Autodesk Fusion 360 part; units mm, degrees
(part 3 of 3)
  spline S32 degree 5 poles (-6.114, -23.4187) (-6.116, -23.4266) (-6.12, -23.4424) (-6.1254, -23.4662) (-6.1316, -23.4981) (-6.138, -23.5383) (-6.1434, -23.5788) (-6.1482, -23.6193) (-6.1527, -23.6599) (-6.157, -23.7006) (-6.1611, -23.7414) (-6.1648, -23.7822) (-6.1682, -23.8231) (-6.1711, -23.864) (-6.1735, -23.9051) (-6.1755, -23.9463) (-6.1771, -23.9875) (-6.1784, -24.0288) (-6.1795, -24.0701) (-6.1802, -24.1115) (-6.1807, -24.1529) (-6.181, -24.1944) (-6.1809, -24.2359) (-6.1806, -24.2775) (-6.18, -24.3191) (-6.1791, -24.3608) (-6.178, -24.4025) (-6.1765, -24.4442) (-6.1749, -24.486) (-6.173, -24.5279) (-6.1709, -24.5697) (-6.1685, -24.6116) (-6.1659, -24.6535) (-6.1631, -24.6955) (-6.16, -24.7375) (-6.1568, -24.7795) (-6.1532, -24.8215) (-6.1495, -24.8636) (-6.1456, -24.9057) (-6.1414, -24.9479) (-6.1371, -24.99) (-6.1325, -25.0322) (-6.1277, -25.0744) (-6.1227, -25.1166) (-6.1175, -25.1589) (-6.1121, -25.2012) (-6.1065, -25.2435) (-6.1007, -25.2858) (-6.0947, -25.3281) (-6.0886, -25.3705) (-6.0822, -25.4128) (-6.0756, -25.4552) (-6.0689, -25.4976) (-6.0619, -25.5401) (-6.0548, -25.5825) (-6.0475, -25.6249) (-6.04, -25.6674) (-6.0323, -25.7099) (-6.0244, -25.7524) (-6.0164, -25.7949) (-6.0081, -25.8374) (-5.9997, -25.88) (-5.9911, -25.9225) (-5.9824, -25.9651) (-5.9734, -26.0076) (-5.9643, -26.0502) (-5.9551, -26.0928) (-5.9456, -26.1354) (-5.936, -26.178) (-5.9262, -26.2206) (-5.9162, -26.2632) (-5.9081, -26.2973) (-5.9019, -26.3229) (-5.8978, -26.3399) (-5.8957, -26.3484) knots 0 0 0 0 0 0 0.01428571 0.02857143 0.04285714 0.05714286 0.07142857 0.08571429 0.1 0.11428571 0.12857143 0.14285714 0.15714286 0.17142857 0.18571429 0.2 0.21428571 0.22857143 0.24285714 0.25714286 0.27142857 0.28571429 0.3 0.31428571 0.32857143 0.34285714 0.35714286 0.37142857 0.38571429 0.4 0.41428571 0.42857143 0.44285714 0.45714286 0.47142857 0.48571429 0.5 0.51428571 0.52857143 0.54285714 0.55714286 0.57142857 0.58571429 0.6 0.61428571 0.62857143 0.64285714 0.65714286 0.67142857 0.68571429 0.7 0.71428571 0.72857143 0.74285714 0.75714286 0.77142857 0.78571429 0.8 0.81428571 0.82857143 0.84285714 0.85714286 0.87142857 0.88571429 0.9 0.91428571 0.92857143 0.94285714 0.95714286 0.97142857 0.98571429 1 1 1 1 1 1
  arc A66 (-5.8957, -26.3484) -> (-4.2178, -26.6685) centre (0, 0) ccw
  spline S33 degree 5 poles (-2.9364, -24.0249) (-2.9374, -24.033) (-2.9395, -24.0491) (-2.9433, -24.0732) (-2.9493, -24.1052) (-2.9581, -24.1449) (-2.9679, -24.1845) (-2.9784, -24.224) (-2.9891, -24.2634) (-3.0001, -24.3028) (-3.0114, -24.3422) (-3.0229, -24.3815) (-3.0348, -24.4208) (-3.0472, -24.46) (-3.0601, -24.499) (-3.0734, -24.538) (-3.087, -24.577) (-3.101, -24.6158) (-3.1153, -24.6546) (-3.1298, -24.6934) (-3.1446, -24.7321) (-3.1596, -24.7708) (-3.1749, -24.8094) (-3.1905, -24.8479) (-3.2064, -24.8864) (-3.2226, -24.9248) (-3.239, -24.9631) (-3.2557, -25.0014) (-3.2726, -25.0397) (-3.2898, -25.0779) (-3.3072, -25.116) (-3.3248, -25.1541) (-3.3426, -25.1921) (-3.3607, -25.2301) (-3.379, -25.268) (-3.3975, -25.3058) (-3.4163, -25.3436) (-3.4352, -25.3814) (-3.4544, -25.4191) (-3.4738, -25.4567) (-3.4934, -25.4943) (-3.5131, -25.5319) (-3.5331, -25.5694) (-3.5533, -25.6068) (-3.5737, -25.6442) (-3.5943, -25.6815) (-3.615, -25.7187) (-3.636, -25.7559) (-3.6571, -25.7931) (-3.6785, -25.8302) (-3.7, -25.8673) (-3.7217, -25.9043) (-3.7436, -25.9412) (-3.7657, -25.9781) (-3.7879, -26.0149) (-3.8104, -26.0517) (-3.833, -26.0884) (-3.8558, -26.1251) (-3.8787, -26.1617) (-3.9019, -26.1983) (-3.9252, -26.2348) (-3.9486, -26.2712) (-3.9723, -26.3076) (-3.9961, -26.344) (-4.0201, -26.3802) (-4.0442, -26.4165) (-4.0685, -26.4527) (-4.093, -26.4888) (-4.1176, -26.5248) (-4.1424, -26.5608) (-4.1674, -26.5968) (-4.1875, -26.6255) (-4.2026, -26.647) (-4.2127, -26.6614) (-4.2178, -26.6685) knots 0 0 0 0 0 0 0.01428571 0.02857143 0.04285714 0.05714286 0.07142857 0.08571429 0.1 0.11428571 0.12857143 0.14285714 0.15714286 0.17142857 0.18571429 0.2 0.21428571 0.22857143 0.24285714 0.25714286 0.27142857 0.28571429 0.3 0.31428571 0.32857143 0.34285714 0.35714286 0.37142857 0.38571429 0.4 0.41428571 0.42857143 0.44285714 0.45714286 0.47142857 0.48571429 0.5 0.51428571 0.52857143 0.54285714 0.55714286 0.57142857 0.58571429 0.6 0.61428571 0.62857143 0.64285714 0.65714286 0.67142857 0.68571429 0.7 0.71428571 0.72857143 0.74285714 0.75714286 0.77142857 0.78571429 0.8 0.81428571 0.82857143 0.84285714 0.85714286 0.87142857 0.88571429 0.9 0.91428571 0.92857143 0.94285714 0.95714286 0.97142857 0.98571429 1 1 1 1 1 1
  line L33 (-2.9364, -24.0249) -> (-2.8541, -23.3538)
  arc A67 (-1.7825, -22.4786) -> (-2.8541, -23.3538) centre (-1.8615, -23.4755) ccw
  arc A68 (-1.7825, -22.4786) -> (-1.0489, -22.5248) centre (0, 0) ccw
  arc A69 (-0.0954, -23.5274) -> (-1.0489, -22.5248) centre (-1.0954, -23.5237) ccw
  line L34 (-0.0954, -23.5274) -> (-0.0979, -24.2035)
  spline S34 degree 5 poles (-0.0979, -24.2035) (-0.0979, -24.2116) (-0.0978, -24.2279) (-0.0971, -24.2523) (-0.0952, -24.2848) (-0.0914, -24.3253) (-0.0866, -24.3658) (-0.0812, -24.4063) (-0.0755, -24.4467) (-0.0695, -24.4872) (-0.0633, -24.5277) (-0.0568, -24.5682) (-0.0498, -24.6086) (-0.0425, -24.649) (-0.0346, -24.6894) (-0.0263, -24.7297) (-0.0176, -24.7701) (-0.0086, -24.8104) (0.0007, -24.8507) (0.0102, -24.891) (0.02, -24.9312) (0.0301, -24.9714) (0.0405, -25.0117) (0.0511, -25.0518) (0.0621, -25.092) (0.0733, -25.1321) (0.0848, -25.1722) (0.0965, -25.2123) (0.1085, -25.2524) (0.1208, -25.2924) (0.1332, -25.3324) (0.1459, -25.3724) (0.1589, -25.4124) (0.172, -25.4523) (0.1855, -25.4922) (0.1991, -25.5321) (0.2129, -25.572) (0.227, -25.6118) (0.2413, -25.6516) (0.2558, -25.6914) (0.2705, -25.7311) (0.2854, -25.7709) (0.3006, -25.8105) (0.3159, -25.8502) (0.3314, -25.8898) (0.3472, -25.9294) (0.3631, -25.969) (0.3792, -26.0086) (0.3956, -26.0481) (0.4121, -26.0876) (0.4288, -26.127) (0.4457, -26.1664) (0.4628, -26.2058) (0.4801, -26.2452) (0.4975, -26.2845) (0.5152, -26.3238) (0.533, -26.3631) (0.551, -26.4023) (0.5692, -26.4415) (0.5876, -26.4807) (0.6061, -26.5199) (0.6248, -26.559) (0.6437, -26.598) (0.6628, -26.6371) (0.6821, -26.6761) (0.7015, -26.715) (0.721, -26.754) (0.7408, -26.7929) (0.7607, -26.8318) (0.7808, -26.8706) (0.8011, -26.9094) (0.8174, -26.9404) (0.8297, -26.9636) (0.838, -26.9791) (0.8421, -26.9869) knots 0 0 0 0 0 0 0.01428571 0.02857143 0.04285714 0.05714286 0.07142857 0.08571429 0.1 0.11428571 0.12857143 0.14285714 0.15714286 0.17142857 0.18571429 0.2 0.21428571 0.22857143 0.24285714 0.25714286 0.27142857 0.28571429 0.3 0.31428571 0.32857143 0.34285714 0.35714286 0.37142857 0.38571429 0.4 0.41428571 0.42857143 0.44285714 0.45714286 0.47142857 0.48571429 0.5 0.51428571 0.52857143 0.54285714 0.55714286 0.57142857 0.58571429 0.6 0.61428571 0.62857143 0.64285714 0.65714286 0.67142857 0.68571429 0.7 0.71428571 0.72857143 0.74285714 0.75714286 0.77142857 0.78571429 0.8 0.81428571 0.82857143 0.84285714 0.85714286 0.87142857 0.88571429 0.9 0.91428571 0.92857143 0.94285714 0.95714286 0.97142857 0.98571429 1 1 1 1 1 1
  arc A70 (0.8421, -26.9869) -> (2.5469, -26.8796) centre (0, 0) ccw
  spline S35 degree 5 poles (3.1306, -24.0004) (3.1317, -24.0084) (3.1336, -24.0246) (3.136, -24.0489) (3.1381, -24.0813) (3.1394, -24.122) (3.1398, -24.1628) (3.1395, -24.2036) (3.1388, -24.2445) (3.138, -24.2854) (3.1369, -24.3264) (3.1355, -24.3673) (3.1337, -24.4083) (3.1315, -24.4493) (3.1287, -24.4904) (3.1256, -24.5314) (3.122, -24.5725) (3.1181, -24.6137) (3.1139, -24.6548) (3.1095, -24.696) (3.1048, -24.7371) (3.0999, -24.7783) (3.0946, -24.8195) (3.0891, -24.8607) (3.0833, -24.9019) (3.0772, -24.9431) (3.0708, -24.9844) (3.0642, -25.0256) (3.0573, -25.0669) (3.0502, -25.1081) (3.0428, -25.1494) (3.0352, -25.1907) (3.0274, -25.2319) (3.0193, -25.2732) (3.011, -25.3145) (3.0025, -25.3557) (2.9938, -25.397) (2.9848, -25.4383) (2.9756, -25.4796) (2.9662, -25.5209) (2.9566, -25.5621) (2.9468, -25.6034) (2.9367, -25.6447) (2.9265, -25.686) (2.916, -25.7272) (2.9054, -25.7685) (2.8945, -25.8098) (2.8835, -25.851) (2.8722, -25.8923) (2.8608, -25.9335) (2.8492, -25.9747) (2.8373, -26.016) (2.8253, -26.0572) (2.8131, -26.0984) (2.8007, -26.1396) (2.7881, -26.1808) (2.7754, -26.222) (2.7624, -26.2632) (2.7493, -26.3044) (2.736, -26.3456) (2.7225, -26.3867) (2.7088, -26.4279) (2.695, -26.469) (2.6809, -26.5101) (2.6667, -26.5512) (2.6523, -26.5923) (2.6378, -26.6334) (2.6231, -26.6745) (2.6082, -26.7155) (2.5931, -26.7566) (2.5779, -26.7976) (2.5656, -26.8304) (2.5563, -26.855) (2.55, -26.8714) (2.5469, -26.8796) knots 0 0 0 0 0 0 0.01428571 0.02857143 0.04285714 0.05714286 0.07142857 0.08571429 0.1 0.11428571 0.12857143 0.14285714 0.15714286 0.17142857 0.18571429 0.2 0.21428571 0.22857143 0.24285714 0.25714286 0.27142857 0.28571429 0.3 0.31428571 0.32857143 0.34285714 0.35714286 0.37142857 0.38571429 0.4 0.41428571 0.42857143 0.44285714 0.45714286 0.47142857 0.48571429 0.5 0.51428571 0.52857143 0.54285714 0.55714286 0.57142857 0.58571429 0.6 0.61428571 0.62857143 0.64285714 0.65714286 0.67142857 0.68571429 0.7 0.71428571 0.72857143 0.74285714 0.75714286 0.77142857 0.78571429 0.8 0.81428571 0.82857143 0.84285714 0.85714286 0.87142857 0.88571429 0.9 0.91428571 0.92857143 0.94285714 0.95714286 0.97142857 0.98571429 1 1 1 1 1 1
  line L35 (3.1306, -24.0004) -> (3.0434, -23.3299)
  arc A71 (3.8637, -22.2157) -> (3.0434, -23.3299) centre (4.0351, -23.2009) ccw
  arc A72 (3.8637, -22.2157) -> (4.5857, -22.078) centre (0, 0) ccw
  arc A73 (5.7586, -22.8119) -> (4.5857, -22.078) centre (4.7891, -23.0571) ccw
  line L36 (5.7586, -22.8119) -> (5.9243, -23.4674)
  spline S36 degree 5 poles (5.9243, -23.4674) (5.9263, -23.4753) (5.9305, -23.4911) (5.9372, -23.5145) (5.9472, -23.5455) (5.9609, -23.5838) (5.9756, -23.6218) (5.9909, -23.6597) (6.0066, -23.6975) (6.0224, -23.7352) (6.0385, -23.7728) (6.0549, -23.8104) (6.0716, -23.8479) (6.0888, -23.8852) (6.1065, -23.9223) (6.1246, -23.9594) (6.143, -23.9963) (6.1618, -24.0331) (6.1808, -24.0698) (6.2, -24.1064) (6.2195, -24.143) (6.2393, -24.1794) (6.2593, -24.2158) (6.2797, -24.2521) (6.3002, -24.2882) (6.3211, -24.3243) (6.3422, -24.3603) (6.3636, -24.3962) (6.3851, -24.432) (6.4069, -24.4678) (6.429, -24.5034) (6.4512, -24.539) (6.4737, -24.5745) (6.4964, -24.6099) (6.5193, -24.6452) (6.5424, -24.6805) (6.5657, -24.7156) (6.5893, -24.7507) (6.613, -24.7857) (6.637, -24.8206) (6.6611, -24.8555) (6.6854, -24.8902) (6.7099, -24.9249) (6.7347, -24.9595) (6.7596, -24.994) (6.7847, -25.0285) (6.8099, -25.0629) (6.8354, -25.0971) (6.861, -25.1314) (6.8869, -25.1655) (6.9129, -25.1996) (6.939, -25.2335) (6.9654, -25.2674) (6.9919, -25.3013) (7.0186, -25.335) (7.0455, -25.3687) (7.0725, -25.4023) (7.0997, -25.4358) (7.1271, -25.4693) (7.1546, -25.5027) (7.1823, -25.5359) (7.2102, -25.5692) (7.2382, -25.6023) (7.2664, -25.6354) (7.2947, -25.6684) (7.3232, -25.7013) (7.3518, -25.7341) (7.3806, -25.7669) (7.4096, -25.7996) (7.4387, -25.8322) (7.468, -25.8648) (7.4915, -25.8907) (7.5092, -25.9102) (7.5211, -25.9231) (7.527, -25.9296) knots 0 0 0 0 0 0 0.01428571 0.02857143 0.04285714 0.05714286 0.07142857 0.08571429 0.1 0.11428571 0.12857143 0.14285714 0.15714286 0.17142857 0.18571429 0.2 0.21428571 0.22857143 0.24285714 0.25714286 0.27142857 0.28571429 0.3 0.31428571 0.32857143 0.34285714 0.35714286 0.37142857 0.38571429 0.4 0.41428571 0.42857143 0.44285714 0.45714286 0.47142857 0.48571429 0.5 0.51428571 0.52857143 0.54285714 0.55714286 0.57142857 0.58571429 0.6 0.61428571 0.62857143 0.64285714 0.65714286 0.67142857 0.68571429 0.7 0.71428571 0.72857143 0.74285714 0.75714286 0.77142857 0.78571429 0.8 0.81428571 0.82857143 0.84285714 0.85714286 0.87142857 0.88571429 0.9 0.91428571 0.92857143 0.94285714 0.95714286 0.97142857 0.98571429 1 1 1 1 1 1
  arc A74 (7.527, -25.9296) -> (9.1516, -25.4017) centre (0, 0) ccw
  spline S37 degree 5 poles (9.0009, -22.4678) (9.0039, -22.4754) (9.0098, -22.4905) (9.0182, -22.5135) (9.0283, -22.5444) (9.0397, -22.5834) (9.0502, -22.6229) (9.06, -22.6625) (9.0696, -22.7022) (9.0789, -22.7421) (9.0881, -22.782) (9.0969, -22.822) (9.1054, -22.8621) (9.1134, -22.9024) (9.1209, -22.9429) (9.1281, -22.9834) (9.1349, -23.0241) (9.1413, -23.0649) (9.1475, -23.1058) (9.1535, -23.1468) (9.1592, -23.1878) (9.1646, -23.2289) (9.1698, -23.2701) (9.1747, -23.3114) (9.1793, -23.3528) (9.1836, -23.3942) (9.1877, -23.4358) (9.1915, -23.4774) (9.1951, -23.519) (9.1985, -23.5608) (9.2016, -23.6026) (9.2045, -23.6444) (9.2072, -23.6863) (9.2097, -23.7283) (9.2119, -23.7704) (9.2139, -23.8125) (9.2157, -23.8546) (9.2173, -23.8968) (9.2186, -23.9391) (9.2198, -23.9814) (9.2207, -24.0238) (9.2215, -24.0662) (9.222, -24.1087) (9.2224, -24.1512) (9.2225, -24.1938) (9.2225, -24.2364) (9.2222, -24.2791) (9.2218, -24.3218) (9.2211, -24.3645) (9.2203, -24.4073) (9.2193, -24.4501) (9.2181, -24.493) (9.2167, -24.5359) (9.2151, -24.5789) (9.2134, -24.6219) (9.2114, -24.6649) (9.2093, -24.708) (9.207, -24.7511) (9.2045, -24.7943) (9.2019, -24.8375) (9.199, -24.8807) (9.196, -24.9239) (9.1929, -24.9672) (9.1895, -25.0105) (9.186, -25.0539) (9.1823, -25.0973) (9.1784, -25.1407) (9.1743, -25.1841) (9.1701, -25.2276) (9.1658, -25.2711) (9.1612, -25.3146) (9.1574, -25.3494) (9.1545, -25.3756) (9.1526, -25.393) (9.1516, -25.4017) knots 0 0 0 0 0 0 0.01428571 0.02857143 0.04285714 0.05714286 0.07142857 0.08571429 0.1 0.11428571 0.12857143 0.14285714 0.15714286 0.17142857 0.18571429 0.2 0.21428571 0.22857143 0.24285714 0.25714286 0.27142857 0.28571429 0.3 0.31428571 0.32857143 0.34285714 0.35714286 0.37142857 0.38571429 0.4 0.41428571 0.42857143 0.44285714 0.45714286 0.47142857 0.48571429 0.5 0.51428571 0.52857143 0.54285714 0.55714286 0.57142857 0.58571429 0.6 0.61428571 0.62857143 0.64285714 0.65714286 0.67142857 0.68571429 0.7 0.71428571 0.72857143 0.74285714 0.75714286 0.77142857 0.78571429 0.8 0.81428571 0.82857143 0.84285714 0.85714286 0.87142857 0.88571429 0.9 0.91428571 0.92857143 0.94285714 0.95714286 0.97142857 0.98571429 1 1 1 1 1 1
  line L37 (9.0009, -22.4678) -> (8.7497, -21.84)
  arc A75 (9.2672, -20.5569) -> (8.7497, -21.84) centre (9.6782, -21.4685) ccw
  arc A76 (9.2672, -20.5569) -> (9.9322, -20.2439) centre (0, 0) ccw
  arc A77 (11.2508, -20.6632) -> (9.9322, -20.2439) centre (10.3727, -21.1417) ccw
  line L38 (11.2508, -20.6632) -> (11.5743, -21.2568)
  spline S38 degree 5 poles (11.5743, -21.2568) (11.5782, -21.264) (11.5862, -21.2782) (11.5985, -21.2992) (11.6159, -21.3267) (11.6387, -21.3604) (11.6624, -21.3936) (11.6867, -21.4265) (11.7112, -21.4592) (11.7359, -21.4918) (11.7609, -21.5243) (11.7861, -21.5566) (11.8116, -21.5887) (11.8375, -21.6205) (11.8639, -21.6521) (11.8906, -21.6835) (11.9176, -21.7147) (11.945, -21.7457) (11.9725, -21.7765) (12.0003, -21.8072) (12.0283, -21.8377) (12.0565, -21.8681) (12.0849, -21.8984) (12.1136, -21.9285) (12.1426, -21.9584) (12.1717, -21.9881) (12.2011, -22.0178) (12.2307, -22.0472) (12.2605, -22.0766) (12.2906, -22.1057) (12.3208, -22.1348) (12.3512, -22.1637) (12.3817, -22.1925) (12.4125, -22.2212) (12.4435, -22.2497) (12.4747, -22.2781) (12.506, -22.3063) (12.5375, -22.3344) (12.5692, -22.3624) (12.6011, -22.3903) (12.6331, -22.418) (12.6653, -22.4457) (12.6977, -22.4732) (12.7303, -22.5005) (12.763, -22.5278) (12.7958, -22.5549) (12.8289, -22.5819) (12.8621, -22.6088) (12.8954, -22.6355) (12.9289, -22.6622) (12.9626, -22.6887) (12.9964, -22.7151) (13.0303, -22.7414) (13.0644, -22.7676) (13.0987, -22.7936) (13.1331, -22.8196) (13.1676, -22.8454) (13.2023, -22.8711) (13.2371, -22.8967) (13.2721, -22.9222) (13.3072, -22.9475) (13.3424, -22.9728) (13.3778, -22.9979) (13.4133, -23.0229) (13.449, -23.0478) (13.4848, -23.0726) (13.5207, -23.0973) (13.5567, -23.1219) (13.5929, -23.1464) (13.6292, -23.1707) (13.6657, -23.195) (13.6949, -23.2143) (13.7169, -23.2287) (13.7316, -23.2383) (13.739, -23.2431) knots 0 0 0 0 0 0 0.01428571 0.02857143 0.04285714 0.05714286 0.07142857 0.08571429 0.1 0.11428571 0.12857143 0.14285714 0.15714286 0.17142857 0.18571429 0.2 0.21428571 0.22857143 0.24285714 0.25714286 0.27142857 0.28571429 0.3 0.31428571 0.32857143 0.34285714 0.35714286 0.37142857 0.38571429 0.4 0.41428571 0.42857143 0.44285714 0.45714286 0.47142857 0.48571429 0.5 0.51428571 0.52857143 0.54285714 0.55714286 0.57142857 0.58571429 0.6 0.61428571 0.62857143 0.64285714 0.65714286 0.67142857 0.68571429 0.7 0.71428571 0.72857143 0.74285714 0.75714286 0.77142857 0.78571429 0.8 0.81428571 0.82857143 0.84285714 0.85714286 0.87142857 0.88571429 0.9 0.91428571 0.92857143 0.94285714 0.95714286 0.97142857 0.98571429 1 1 1 1 1 1
  arc A78 (13.739, -23.2431) -> (15.1812, -22.3278) centre (0, 0) ccw
  spline S39 degree 5 poles (14.3057, -19.5235) (14.3105, -19.5301) (14.3199, -19.5433) (14.3337, -19.5634) (14.3512, -19.5908) (14.372, -19.6259) (14.3919, -19.6614) (14.4113, -19.6974) (14.4305, -19.7335) (14.4494, -19.7697) (14.4682, -19.8061) (14.4867, -19.8427) (14.5049, -19.8795) (14.5227, -19.9165) (14.5401, -19.9538) (14.5571, -19.9913) (14.5737, -20.0291) (14.5901, -20.067) (14.6063, -20.105) (14.6223, -20.1432) (14.638, -20.1815) (14.6535, -20.22) (14.6687, -20.2586) (14.6837, -20.2974) (14.6985, -20.3363) (14.713, -20.3754) (14.7273, -20.4146) (14.7413, -20.454) (14.7552, -20.4934) (14.7688, -20.533) (14.7822, -20.5727) (14.7955, -20.6125) (14.8085, -20.6524) (14.8213, -20.6925) (14.8339, -20.7327) (14.8463, -20.7729) (14.8586, -20.8133) (14.8706, -20.8538) (14.8824, -20.8944) (14.8941, -20.9351) (14.9055, -20.9759) (14.9168, -21.0168) (14.9279, -21.0578) (14.9388, -21.0989) (14.9495, -21.1401) (14.9601, -21.1814) (14.9704, -21.2228) (14.9806, -21.2643) (14.9907, -21.3059) (15.0005, -21.3475) (15.0102, -21.3893) (15.0197, -21.4311) (15.029, -21.473) (15.0382, -21.515) (15.0471, -21.5571) (15.056, -21.5993) (15.0646, -21.6415) (15.0731, -21.6838) (15.0814, -21.7262) (15.0896, -21.7687) (15.0976, -21.8113) (15.1055, -21.8539) (15.1131, -21.8966) (15.1207, -21.9394) (15.128, -21.9823) (15.1352, -22.0252) (15.1423, -22.0683) (15.1491, -22.1113) (15.1559, -22.1545) (15.1625, -22.1977) (15.1689, -22.241) (15.1739, -22.2757) (15.1776, -22.3017) (15.18, -22.3191) (15.1812, -22.3278) knots 0 0 0 0 0 0 0.01428571 0.02857143 0.04285714 0.05714286 0.07142857 0.08571429 0.1 0.11428571 0.12857143 0.14285714 0.15714286 0.17142857 0.18571429 0.2 0.21428571 0.22857143 0.24285714 0.25714286 0.27142857 0.28571429 0.3 0.31428571 0.32857143 0.34285714 0.35714286 0.37142857 0.38571429 0.4 0.41428571 0.42857143 0.44285714 0.45714286 0.47142857 0.48571429 0.5 0.51428571 0.52857143 0.54285714 0.55714286 0.57142857 0.58571429 0.6 0.61428571 0.62857143 0.64285714 0.65714286 0.67142857 0.68571429 0.7 0.71428571 0.72857143 0.74285714 0.75714286 0.77142857 0.78571429 0.8 0.81428571 0.82857143 0.84285714 0.85714286 0.87142857 0.88571429 0.9 0.91428571 0.92857143 0.94285714 0.95714286 0.97142857 0.98571429 1 1 1 1 1 1
  line L39 (14.3057, -19.5235) -> (13.9062, -18.9779)
  arc A79 (14.0883, -17.6064) -> (13.9062, -18.9779) centre (14.7131, -18.3872) ccw
  arc A80 (14.0883, -17.6064) -> (14.6547, -17.1379) centre (0, 0) ccw
  arc A81 (16.036, -17.216) -> (14.6547, -17.1379) centre (15.3046, -17.8979) ccw
  line L40 (16.036, -17.216) -> (16.4971, -17.7106)
  spline S40 degree 5 poles (16.4971, -17.7106) (16.5026, -17.7166) (16.5138, -17.7283) (16.531, -17.7456) (16.5547, -17.768) (16.5852, -17.7949) (16.6164, -17.8212) (16.648, -17.847) (16.6799, -17.8726) (16.712, -17.898) (16.7442, -17.9232) (16.7767, -17.9483) (16.8094, -17.973) (16.8424, -17.9974) (16.8758, -18.0215) (16.9095, -18.0452) (16.9434, -18.0687) (16.9776, -18.0919) (17.012, -18.1149) (17.0465, -18.1377) (17.0812, -18.1604) (17.1161, -18.1828) (17.1512, -18.205) (17.1864, -18.227) (17.2219, -18.2488) (17.2576, -18.2704) (17.2934, -18.2917) (17.3294, -18.3129) (17.3656, -18.3339) (17.4019, -18.3547) (17.4384, -18.3753) (17.475, -18.3958) (17.5118, -18.4161) (17.5487, -18.4362) (17.5858, -18.4561) (17.6231, -18.4758) (17.6605, -18.4954) (17.698, -18.5148) (17.7356, -18.534) (17.7734, -18.5531) (17.8114, -18.572) (17.8494, -18.5907) (17.8876, -18.6093) (17.926, -18.6277) (17.9644, -18.646) (18.003, -18.6641) (18.0417, -18.682) (18.0805, -18.6998) (18.1195, -18.7174) (18.1586, -18.7349) (18.1978, -18.7522) (18.2371, -18.7694) (18.2765, -18.7864) (18.316, -18.8033) (18.3557, -18.82) (18.3955, -18.8366) (18.4353, -18.853) (18.4753, -18.8693) (18.5154, -18.8854) (18.5556, -18.9014) (18.5959, -18.9172) (18.6364, -18.9329) (18.6769, -18.9485) (18.7175, -18.9639) (18.7582, -18.9791) (18.7991, -18.9942) (18.84, -19.0092) (18.881, -19.0241) (18.9221, -19.0388) (18.9634, -19.0533) (19.0047, -19.0677) (19.0378, -19.0792) (19.0627, -19.0877) (19.0793, -19.0933) (19.0876, -19.0961) knots 0 0 0 0 0 0 0.01428571 0.02857143 0.04285714 0.05714286 0.07142857 0.08571429 0.1 0.11428571 0.12857143 0.14285714 0.15714286 0.17142857 0.18571429 0.2 0.21428571 0.22857143 0.24285714 0.25714286 0.27142857 0.28571429 0.3 0.31428571 0.32857143 0.34285714 0.35714286 0.37142857 0.38571429 0.4 0.41428571 0.42857143 0.44285714 0.45714286 0.47142857 0.48571429 0.5 0.51428571 0.52857143 0.54285714 0.55714286 0.57142857 0.58571429 0.6 0.61428571 0.62857143 0.64285714 0.65714286 0.67142857 0.68571429 0.7 0.71428571 0.72857143 0.74285714 0.75714286 0.77142857 0.78571429 0.8 0.81428571 0.82857143 0.84285714 0.85714286 0.87142857 0.88571429 0.9 0.91428571 0.92857143 0.94285714 0.95714286 0.97142857 0.98571429 1 1 1 1 1 1
  arc A82 (19.0876, -19.0961) -> (20.257, -17.8509) centre (0, 0) ccw
  spline S41 degree 5 poles (18.7115, -15.3525) (18.7178, -15.3576) (18.7303, -15.3681) (18.7486, -15.3842) (18.7724, -15.4063) (18.8012, -15.4351) (18.8294, -15.4646) (18.8571, -15.4946) (18.8846, -15.5248) (18.912, -15.5552) (18.9392, -15.5858) (18.9663, -15.6166) (18.993, -15.6477) (19.0195, -15.6791) (19.0456, -15.7109) (19.0714, -15.7431) (19.0969, -15.7755) (19.1222, -15.8081) (19.1473, -15.8409) (19.1723, -15.874) (19.1971, -15.9072) (19.2216, -15.9406) (19.246, -15.9742) (19.2702, -16.008) (19.2942, -16.0421) (19.3179, -16.0763) (19.3415, -16.1107) (19.3649, -16.1453) (19.3881, -16.1801) (19.4112, -16.2151) (19.4341, -16.2502) (19.4568, -16.2854) (19.4793, -16.3209) (19.5017, -16.3565) (19.5239, -16.3923) (19.5459, -16.4282) (19.5678, -16.4643) (19.5895, -16.5005) (19.6111, -16.5369) (19.6325, -16.5734) (19.6537, -16.6101) (19.6748, -16.6469) (19.6958, -16.6839) (19.7166, -16.7209) (19.7372, -16.7582) (19.7577, -16.7956) (19.778, -16.8331) (19.7982, -16.8707) (19.8182, -16.9085) (19.8381, -16.9464) (19.8579, -16.9844) (19.8775, -17.0225) (19.8969, -17.0608) (19.9163, -17.0992) (19.9354, -17.1378) (19.9545, -17.1764) (19.9734, -17.2152) (19.9921, -17.2541) (20.0107, -17.2931) (20.0292, -17.3322) (20.0475, -17.3714) (20.0657, -17.4108) (20.0838, -17.4502) (20.1017, -17.4898) (20.1195, -17.5295) (20.1372, -17.5693) (20.1547, -17.6092) (20.1721, -17.6492) (20.1893, -17.6893) (20.2064, -17.7296) (20.2234, -17.7699) (20.2369, -17.8023) (20.247, -17.8266) (20.2536, -17.8428) (20.257, -17.8509) knots 0 0 0 0 0 0 0.01428571 0.02857143 0.04285714 0.05714286 0.07142857 0.08571429 0.1 0.11428571 0.12857143 0.14285714 0.15714286 0.17142857 0.18571429 0.2 0.21428571 0.22857143 0.24285714 0.25714286 0.27142857 0.28571429 0.3 0.31428571 0.32857143 0.34285714 0.35714286 0.37142857 0.38571429 0.4 0.41428571 0.42857143 0.44285714 0.45714286 0.47142857 0.48571429 0.5 0.51428571 0.52857143 0.54285714 0.55714286 0.57142857 0.58571429 0.6 0.61428571 0.62857143 0.64285714 0.65714286 0.67142857 0.68571429 0.7 0.71428571 0.72857143 0.74285714 0.75714286 0.77142857 0.78571429 0.8 0.81428571 0.82857143 0.84285714 0.85714286 0.87142857 0.88571429 0.9 0.91428571 0.92857143 0.94285714 0.95714286 0.97142857 0.98571429 1 1 1 1 1 1
  line L41 (18.7115, -15.3525) -> (18.189, -14.9234)
  arc A83 (18.0243, -13.5496) -> (18.189, -14.9234) centre (18.8236, -14.1505) ccw
  arc A84 (18.0243, -13.5496) -> (18.4563, -12.955) centre (0, 0) ccw
  arc A85 (19.8137, -12.6872) -> (18.4563, -12.955) centre (19.2748, -13.5295) ccw
  line L42 (19.8137, -12.6872) -> (20.3832, -13.0515)
  spline S42 degree 5 poles (20.3832, -13.0515) (20.3901, -13.0559) (20.4039, -13.0645) (20.4248, -13.077) (20.4533, -13.0928) (20.4895, -13.1113) (20.5263, -13.129) (20.5634, -13.1461) (20.6006, -13.1629) (20.638, -13.1796) (20.6755, -13.196) (20.7132, -13.2122) (20.751, -13.228) (20.7891, -13.2435) (20.8274, -13.2585) (20.8659, -13.2731) (20.9046, -13.2873) (20.9435, -13.3013) (20.9825, -13.3151) (21.0216, -13.3286) (21.0609, -13.3419) (21.1002, -13.3549) (21.1397, -13.3677) (21.1794, -13.3803) (21.2191, -13.3926) (21.259, -13.4046) (21.2991, -13.4164) (21.3392, -13.4279) (21.3795, -13.4393) (21.4198, -13.4504) (21.4603, -13.4613) (21.5009, -13.472) (21.5415, -13.4825) (21.5823, -13.4928) (21.6232, -13.5028) (21.6642, -13.5127) (21.7052, -13.5224) (21.7464, -13.5318) (21.7877, -13.5411) (21.829, -13.5501) (21.8705, -13.559) (21.912, -13.5677) (21.9536, -13.5762) (21.9953, -13.5845) (22.0371, -13.5926) (22.079, -13.6006) (22.1209, -13.6083) (22.163, -13.6159) (22.2051, -13.6233) (22.2473, -13.6305) (22.2895, -13.6375) (22.3319, -13.6444) (22.3743, -13.651) (22.4168, -13.6575) (22.4594, -13.6639) (22.502, -13.67) (22.5447, -13.676) (22.5875, -13.6818) (22.6303, -13.6875) (22.6733, -13.693) (22.7162, -13.6983) (22.7593, -13.7034) (22.8024, -13.7084) (22.8456, -13.7132) (22.8888, -13.7179) (22.9321, -13.7224) (22.9755, -13.7267) (23.0189, -13.7309) (23.0624, -13.7349) (23.106, -13.7387) (23.1496, -13.7424) (23.1845, -13.7452) (23.2107, -13.7473) (23.2282, -13.7486) (23.237, -13.7493) knots 0 0 0 0 0 0 0.01428571 0.02857143 0.04285714 0.05714286 0.07142857 0.08571429 0.1 0.11428571 0.12857143 0.14285714 0.15714286 0.17142857 0.18571429 0.2 0.21428571 0.22857143 0.24285714 0.25714286 0.27142857 0.28571429 0.3 0.31428571 0.32857143 0.34285714 0.35714286 0.37142857 0.38571429 0.4 0.41428571 0.42857143 0.44285714 0.45714286 0.47142857 0.48571429 0.5 0.51428571 0.52857143 0.54285714 0.55714286 0.57142857 0.58571429 0.6 0.61428571 0.62857143 0.64285714 0.65714286 0.67142857 0.68571429 0.7 0.71428571 0.72857143 0.74285714 0.75714286 0.77142857 0.78571429 0.8 0.81428571 0.82857143 0.84285714 0.85714286 0.87142857 0.88571429 0.9 0.91428571 0.92857143 0.94285714 0.95714286 0.97142857 0.98571429 1 1 1 1 1 1
  arc A86 (23.237, -13.7493) -> (24.0599, -12.2524) centre (0, 0) ccw
  spline S43 degree 5 poles (21.9417, -10.2168) (21.949, -10.2202) (21.9637, -10.2272) (21.9855, -10.2382) (22.014, -10.2538) (22.0491, -10.2745) (22.0837, -10.2961) (22.118, -10.3182) (22.1522, -10.3406) (22.1863, -10.3633) (22.2203, -10.3861) (22.2541, -10.4093) (22.2877, -10.4327) (22.3212, -10.4566) (22.3544, -10.4809) (22.3873, -10.5056) (22.4201, -10.5306) (22.4528, -10.556) (22.4853, -10.5815) (22.5177, -10.6073) (22.5499, -10.6333) (22.582, -10.6596) (22.614, -10.6861) (22.6458, -10.7128) (22.6775, -10.7398) (22.709, -10.7671) (22.7404, -10.7945) (22.7717, -10.8222) (22.8028, -10.8502) (22.8339, -10.8783) (22.8648, -10.9066) (22.8955, -10.9351) (22.9262, -10.9638) (22.9567, -10.9927) (22.9871, -11.0219) (23.0174, -11.0512) (23.0476, -11.0807) (23.0776, -11.1104) (23.1075, -11.1403) (23.1373, -11.1703) (23.167, -11.2006) (23.1966, -11.231) (23.2261, -11.2616) (23.2555, -11.2923) (23.2847, -11.3233) (23.3138, -11.3544) (23.3429, -11.3856) (23.3718, -11.4171) (23.4006, -11.4487) (23.4293, -11.4804) (23.4579, -11.5123) (23.4863, -11.5444) (23.5147, -11.5767) (23.543, -11.6091) (23.5711, -11.6416) (23.5992, -11.6743) (23.6271, -11.7072) (23.6549, -11.7402) (23.6827, -11.7733) (23.7103, -11.8066) (23.7378, -11.84) (23.7652, -11.8736) (23.7925, -11.9074) (23.8197, -11.9412) (23.8468, -11.9753) (23.8738, -12.0094) (23.9007, -12.0437) (23.9275, -12.0782) (23.9542, -12.1127) (23.9808, -12.1474) (24.0073, -12.1823) (24.0284, -12.2103) (24.0442, -12.2313) (24.0547, -12.2454) (24.0599, -12.2524) knots 0 0 0 0 0 0 0.01428571 0.02857143 0.04285714 0.05714286 0.07142857 0.08571429 0.1 0.11428571 0.12857143 0.14285714 0.15714286 0.17142857 0.18571429 0.2 0.21428571 0.22857143 0.24285714 0.25714286 0.27142857 0.28571429 0.3 0.31428571 0.32857143 0.34285714 0.35714286 0.37142857 0.38571429 0.4 0.41428571 0.42857143 0.44285714 0.45714286 0.47142857 0.48571429 0.5 0.51428571 0.52857143 0.54285714 0.55714286 0.57142857 0.58571429 0.6 0.61428571 0.62857143 0.64285714 0.65714286 0.67142857 0.68571429 0.7 0.71428571 0.72857143 0.74285714 0.75714286 0.77142857 0.78571429 0.8 0.81428571 0.82857143 0.84285714 0.85714286 0.87142857 0.88571429 0.9 0.91428571 0.92857143 0.94285714 0.95714286 0.97142857 0.98571429 1 1 1 1 1 1
  line L43 (21.9417, -10.2168) -> (21.3288, -9.9311)
  arc A87 (20.8276, -8.6415) -> (21.3288, -9.9311) centre (21.7513, -9.0247) ccw
  arc A88 (20.8276, -8.6415) -> (21.0982, -7.9581) centre (0, 0) ccw
  arc A89 (22.3464, -7.3611) -> (21.0982, -7.9581) centre (22.0339, -8.311) ccw
  line L44 (22.3464, -7.3611) -> (22.9886, -7.5724)
  spline S44 degree 5 poles (22.9886, -7.5724) (22.9964, -7.5749) (23.0119, -7.5799) (23.0353, -7.5867) (23.0668, -7.5949) (23.1065, -7.6038) (23.1465, -7.6118) (23.1867, -7.6192) (23.2269, -7.6262) (23.2673, -7.633) (23.3077, -7.6396) (23.3482, -7.646) (23.3888, -7.6519) (23.4295, -7.6573) (23.4703, -7.6624) (23.5113, -7.6669) (23.5523, -7.6711) (23.5934, -7.675) (23.6346, -7.6786) (23.6759, -7.682) (23.7172, -7.6851) (23.7586, -7.688) (23.8, -7.6905) (23.8415, -7.6928) (23.8831, -7.6948) (23.9247, -7.6965) (23.9664, -7.698) (24.0082, -7.6992) (24.05, -7.7002) (24.0919, -7.7009) (24.1338, -7.7014) (24.1757, -7.7017) (24.2177, -7.7018) (24.2598, -7.7016) (24.3019, -7.7012) (24.344, -7.7005) (24.3862, -7.6997) (24.4284, -7.6986) (24.4707, -7.6973) (24.513, -7.6958) (24.5554, -7.6941) (24.5977, -7.6922) (24.6402, -7.69) (24.6826, -7.6877) (24.7251, -7.6852) (24.7677, -7.6825) (24.8102, -7.6795) (24.8528, -7.6764) (24.8954, -7.6731) (24.9381, -7.6696) (24.9808, -7.6659) (25.0235, -7.662) (25.0663, -7.6579) (25.109, -7.6536) (25.1518, -7.6492) (25.1947, -7.6445) (25.2375, -7.6397) (25.2804, -7.6347) (25.3233, -7.6295) (25.3662, -7.6242) (25.4092, -7.6186) (25.4522, -7.6129) (25.4952, -7.607) (25.5382, -7.6009) (25.5812, -7.5947) (25.6243, -7.5883) (25.6674, -7.5817) (25.7105, -7.5749) (25.7536, -7.568) (25.7967, -7.5609) (25.8399, -7.5536) (25.8744, -7.5477) (25.9003, -7.5431) (25.9176, -7.5401) (25.9263, -7.5385) knots 0 0 0 0 0 0 0.01428571 0.02857143 0.04285714 0.05714286 0.07142857 0.08571429 0.1 0.11428571 0.12857143 0.14285714 0.15714286 0.17142857 0.18571429 0.2 0.21428571 0.22857143 0.24285714 0.25714286 0.27142857 0.28571429 0.3 0.31428571 0.32857143 0.34285714 0.35714286 0.37142857 0.38571429 0.4 0.41428571 0.42857143 0.44285714 0.45714286 0.47142857 0.48571429 0.5 0.51428571 0.52857143 0.54285714 0.55714286 0.57142857 0.58571429 0.6 0.61428571 0.62857143 0.64285714 0.65714286 0.67142857 0.68571429 0.7 0.71428571 0.72857143 0.74285714 0.75714286 0.77142857 0.78571429 0.8 0.81428571 0.82857143 0.84285714 0.85714286 0.87142857 0.88571429 0.9 0.91428571 0.92857143 0.94285714 0.95714286 0.97142857 0.98571429 1 1 1 1 1 1
  arc A90 (25.9263, -7.5385) -> (26.3511, -5.884) centre (0, 0) ccw
  spline S45 degree 5 poles (23.7931, -4.4391) (23.8011, -4.4406) (23.8171, -4.4438) (23.8409, -4.449) (23.8724, -4.457) (23.9115, -4.4683) (23.9504, -4.4806) (23.9892, -4.4935) (24.0279, -4.5067) (24.0665, -4.5202) (24.1051, -4.5339) (24.1436, -4.5479) (24.182, -4.5622) (24.2204, -4.577) (24.2586, -4.5923) (24.2966, -4.608) (24.3346, -4.6241) (24.3725, -4.6405) (24.4104, -4.6572) (24.4482, -4.6741) (24.4859, -4.6913) (24.5235, -4.7088) (24.561, -4.7265) (24.5985, -4.7445) (24.6359, -4.7627) (24.6732, -4.7813) (24.7105, -4.8001) (24.7477, -4.8192) (24.7848, -4.8384) (24.8218, -4.858) (24.8588, -4.8777) (24.8957, -4.8977) (24.9325, -4.9179) (24.9693, -4.9383) (25.006, -4.9589) (25.0426, -4.9798) (25.0791, -5.0009) (25.1156, -5.0222) (25.152, -5.0437) (25.1884, -5.0654) (25.2247, -5.0873) (25.2609, -5.1094) (25.297, -5.1317) (25.3331, -5.1542) (25.3692, -5.1768) (25.4051, -5.1997) (25.441, -5.2228) (25.4768, -5.246) (25.5126, -5.2695) (25.5483, -5.2931) (25.5839, -5.3169) (25.6195, -5.3409) (25.6549, -5.3651) (25.6904, -5.3894) (25.7257, -5.414) (25.761, -5.4387) (25.7963, -5.4635) (25.8314, -5.4886) (25.8665, -5.5138) (25.9016, -5.5392) (25.9365, -5.5647) (25.9714, -5.5904) (26.0063, -5.6163) (26.0411, -5.6424) (26.0758, -5.6686) (26.1104, -5.6949) (26.145, -5.7215) (26.1795, -5.7482) (26.2139, -5.775) (26.2483, -5.802) (26.2826, -5.8292) (26.31, -5.851) (26.3306, -5.8675) (26.3442, -5.8785) (26.3511, -5.884) knots 0 0 0 0 0 0 0.01428571 0.02857143 0.04285714 0.05714286 0.07142857 0.08571429 0.1 0.11428571 0.12857143 0.14285714 0.15714286 0.17142857 0.18571429 0.2 0.21428571 0.22857143 0.24285714 0.25714286 0.27142857 0.28571429 0.3 0.31428571 0.32857143 0.34285714 0.35714286 0.37142857 0.38571429 0.4 0.41428571 0.42857143 0.44285714 0.45714286 0.47142857 0.48571429 0.5 0.51428571 0.52857143 0.54285714 0.55714286 0.57142857 0.58571429 0.6 0.61428571 0.62857143 0.64285714 0.65714286 0.67142857 0.68571429 0.7 0.71428571 0.72857143 0.74285714 0.75714286 0.77142857 0.78571429 0.8 0.81428571 0.82857143 0.84285714 0.85714286 0.87142857 0.88571429 0.9 0.91428571 0.92857143 0.94285714 0.95714286 0.97142857 0.98571429 1 1 1 1 1 1
  line L45 (23.7931, -4.4391) -> (23.1285, -4.3148)
  arc A91 (22.3224, -3.1904) -> (23.1285, -4.3148) centre (23.3123, -3.3319) ccw
  arc A92 (22.3224, -3.1904) -> (22.4145, -2.4612) centre (0, 0) ccw
  arc A93 (23.4749, -1.5725) -> (22.4145, -2.4612) centre (23.4085, -2.5703) ccw
  line L46 (23.4749, -1.5725) -> (24.1496, -1.6175)
  spline S46 degree 5 poles (24.1496, -1.6175) (24.1577, -1.618) (24.174, -1.6189) (24.1983, -1.6197) (24.2309, -1.6198) (24.2716, -1.6186) (24.3123, -1.6164) (24.353, -1.6135) (24.3938, -1.6103) (24.4345, -1.6069) (24.4753, -1.6032) (24.5161, -1.5993) (24.5569, -1.5949) (24.5977, -1.5901) (24.6385, -1.5848) (24.6793, -1.579) (24.7201, -1.5729) (24.7609, -1.5664) (24.8017, -1.5597) (24.8425, -1.5527) (24.8833, -1.5454) (24.9241, -1.5379) (24.9648, -1.5301) (25.0056, -1.522) (25.0464, -1.5136) (25.0871, -1.5049) (25.1279, -1.496) (25.1686, -1.4867) (25.2094, -1.4773) (25.2501, -1.4676) (25.2908, -1.4577) (25.3315, -1.4475) (25.3722, -1.4371) (25.4129, -1.4265) (25.4536, -1.4156) (25.4942, -1.4045) (25.5349, -1.3932) (25.5755, -1.3816) (25.6161, -1.3698) (25.6568, -1.3579) (25.6973, -1.3457) (25.7379, -1.3333) (25.7785, -1.3207) (25.819, -1.3079) (25.8596, -1.2949) (25.9001, -1.2816) (25.9406, -1.2682) (25.9811, -1.2546) (26.0215, -1.2408) (26.062, -1.2268) (26.1024, -1.2126) (26.1428, -1.1982) (26.1832, -1.1836) (26.2236, -1.1688) (26.2639, -1.1539) (26.3042, -1.1387) (26.3446, -1.1234) (26.3848, -1.1079) (26.4251, -1.0922) (26.4654, -1.0763) (26.5056, -1.0603) (26.5458, -1.044) (26.586, -1.0276) (26.6261, -1.0111) (26.6663, -0.9943) (26.7064, -0.9774) (26.7465, -0.9603) (26.7865, -0.943) (26.8266, -0.9256) (26.8666, -0.908) (26.9066, -0.8902) (26.9386, -0.8758) (26.9625, -0.865) (26.9785, -0.8577) (26.9865, -0.8541) knots 0 0 0 0 0 0 0.01428571 0.02857143 0.04285714 0.05714286 0.07142857 0.08571429 0.1 0.11428571 0.12857143 0.14285714 0.15714286 0.17142857 0.18571429 0.2 0.21428571 0.22857143 0.24285714 0.25714286 0.27142857 0.28571429 0.3 0.31428571 0.32857143 0.34285714 0.35714286 0.37142857 0.38571429 0.4 0.41428571 0.42857143 0.44285714 0.45714286 0.47142857 0.48571429 0.5 0.51428571 0.52857143 0.54285714 0.55714286 0.57142857 0.58571429 0.6 0.61428571 0.62857143 0.64285714 0.65714286 0.67142857 0.68571429 0.7 0.71428571 0.72857143 0.74285714 0.75714286 0.77142857 0.78571429 0.8 0.81428571 0.82857143 0.84285714 0.85714286 0.87142857 0.88571429 0.9 0.91428571 0.92857143 0.94285714 0.95714286 0.97142857 0.98571429 1 1 1 1 1 1
  arc A94 (26.9865, -0.8541) -> (26.9865, 0.8541) centre (0, 0) ccw
  spline S47 degree 5 poles (24.1496, 1.6175) (24.1577, 1.618) (24.174, 1.6189) (24.1983, 1.6197) (24.2309, 1.6198) (24.2716, 1.6186) (24.3123, 1.6164) (24.353, 1.6135) (24.3938, 1.6103) (24.4345, 1.6069) (24.4753, 1.6032) (24.5161, 1.5993) (24.5569, 1.5949) (24.5977, 1.5901) (24.6385, 1.5848) (24.6793, 1.579) (24.7201, 1.5729) (24.7609, 1.5664) (24.8017, 1.5597) (24.8425, 1.5527) (24.8833, 1.5455) (24.9241, 1.5379) (24.9648, 1.5301) (25.0056, 1.522) (25.0464, 1.5136) (25.0871, 1.5049) (25.1279, 1.496) (25.1686, 1.4867) (25.2094, 1.4773) (25.2501, 1.4676) (25.2908, 1.4577) (25.3315, 1.4475) (25.3722, 1.4371) (25.4129, 1.4265) (25.4536, 1.4156) (25.4942, 1.4045) (25.5349, 1.3932) (25.5755, 1.3816) (25.6161, 1.3698) (25.6568, 1.3579) (25.6973, 1.3457) (25.7379, 1.3333) (25.7785, 1.3207) (25.819, 1.3079) (25.8596, 1.2949) (25.9001, 1.2816) (25.9406, 1.2682) (25.9811, 1.2546) (26.0215, 1.2408) (26.062, 1.2268) (26.1024, 1.2126) (26.1428, 1.1982) (26.1832, 1.1836) (26.2236, 1.1688) (26.2639, 1.1539) (26.3042, 1.1387) (26.3446, 1.1234) (26.3848, 1.1079) (26.4251, 1.0922) (26.4654, 1.0763) (26.5056, 1.0603) (26.5458, 1.044) (26.586, 1.0276) (26.6261, 1.0111) (26.6663, 0.9943) (26.7064, 0.9774) (26.7465, 0.9603) (26.7865, 0.943) (26.8266, 0.9256) (26.8666, 0.908) (26.9066, 0.8902) (26.9386, 0.8758) (26.9625, 0.865) (26.9785, 0.8577) (26.9865, 0.8541) knots 0 0 0 0 0 0 0.01428571 0.02857143 0.04285714 0.05714286 0.07142857 0.08571429 0.1 0.11428571 0.12857143 0.14285714 0.15714286 0.17142857 0.18571429 0.2 0.21428571 0.22857143 0.24285714 0.25714286 0.27142857 0.28571429 0.3 0.31428571 0.32857143 0.34285714 0.35714286 0.37142857 0.38571429 0.4 0.41428571 0.42857143 0.44285714 0.45714286 0.47142857 0.48571429 0.5 0.51428571 0.52857143 0.54285714 0.55714286 0.57142857 0.58571429 0.6 0.61428571 0.62857143 0.64285714 0.65714286 0.67142857 0.68571429 0.7 0.71428571 0.72857143 0.74285714 0.75714286 0.77142857 0.78571429 0.8 0.81428571 0.82857143 0.84285714 0.85714286 0.87142857 0.88571429 0.9 0.91428571 0.92857143 0.94285714 0.95714286 0.97142857 0.98571429 1 1 1 1 1 1
  line L47 (24.1496, 1.6175) -> (23.4749, 1.5725)
  arc A95 (22.4145, 2.4612) -> (23.4749, 1.5725) centre (23.4085, 2.5703) ccw
  arc A96 (22.4145, 2.4612) -> (22.3224, 3.1904) centre (0, 0) ccw
  arc A97 (23.1285, 4.3148) -> (22.3224, 3.1904) centre (23.3123, 3.3319) ccw
  line L48 (23.1285, 4.3148) -> (23.7931, 4.4391)
  spline S48 degree 5 poles (23.7931, 4.4391) (23.8011, 4.4406) (23.8171, 4.4438) (23.8409, 4.449) (23.8724, 4.457) (23.9115, 4.4683) (23.9504, 4.4806) (23.9892, 4.4935) (24.0279, 4.5067) (24.0665, 4.5202) (24.1051, 4.5339) (24.1436, 4.5479) (24.182, 4.5622) (24.2204, 4.577) (24.2586, 4.5923) (24.2966, 4.6081) (24.3346, 4.6241) (24.3725, 4.6405) (24.4104, 4.6572) (24.4482, 4.6741) (24.4859, 4.6913) (24.5235, 4.7088) (24.561, 4.7265) (24.5985, 4.7445) (24.6359, 4.7627) (24.6732, 4.7813) (24.7105, 4.8001) (24.7477, 4.8192) (24.7848, 4.8384) (24.8218, 4.858) (24.8588, 4.8777) (24.8957, 4.8977) (24.9325, 4.9179) (24.9693, 4.9383) (25.006, 4.9589) (25.0426, 4.9798) (25.0791, 5.0009) (25.1156, 5.0222) (25.152, 5.0437) (25.1884, 5.0654) (25.2247, 5.0873) (25.2609, 5.1094) (25.297, 5.1317) (25.3331, 5.1542) (25.3692, 5.1768) (25.4051, 5.1997) (25.441, 5.2228) (25.4768, 5.246) (25.5126, 5.2695) (25.5483, 5.2931) (25.5839, 5.3169) (25.6195, 5.3409) (25.6549, 5.3651) (25.6904, 5.3894) (25.7257, 5.414) (25.761, 5.4387) (25.7963, 5.4635) (25.8314, 5.4886) (25.8665, 5.5138) (25.9016, 5.5392) (25.9365, 5.5647) (25.9714, 5.5904) (26.0063, 5.6163) (26.0411, 5.6424) (26.0758, 5.6686) (26.1104, 5.6949) (26.145, 5.7215) (26.1795, 5.7482) (26.2139, 5.775) (26.2483, 5.802) (26.2826, 5.8292) (26.31, 5.851) (26.3306, 5.8675) (26.3442, 5.8785) (26.3511, 5.884) knots 0 0 0 0 0 0 0.01428571 0.02857143 0.04285714 0.05714286 0.07142857 0.08571429 0.1 0.11428571 0.12857143 0.14285714 0.15714286 0.17142857 0.18571429 0.2 0.21428571 0.22857143 0.24285714 0.25714286 0.27142857 0.28571429 0.3 0.31428571 0.32857143 0.34285714 0.35714286 0.37142857 0.38571429 0.4 0.41428571 0.42857143 0.44285714 0.45714286 0.47142857 0.48571429 0.5 0.51428571 0.52857143 0.54285714 0.55714286 0.57142857 0.58571429 0.6 0.61428571 0.62857143 0.64285714 0.65714286 0.67142857 0.68571429 0.7 0.71428571 0.72857143 0.74285714 0.75714286 0.77142857 0.78571429 0.8 0.81428571 0.82857143 0.84285714 0.85714286 0.87142857 0.88571429 0.9 0.91428571 0.92857143 0.94285714 0.95714286 0.97142857 0.98571429 1 1 1 1 1 1
  arc A98 (26.3511, 5.884) -> (25.9263, 7.5385) centre (0, 0) ccw
  spline S49 degree 5 poles (22.9886, 7.5724) (22.9964, 7.5749) (23.0119, 7.5799) (23.0353, 7.5867) (23.0668, 7.5949) (23.1065, 7.6039) (23.1465, 7.6118) (23.1867, 7.6192) (23.2269, 7.6262) (23.2673, 7.633) (23.3077, 7.6396) (23.3482, 7.646) (23.3888, 7.6519) (23.4295, 7.6573) (23.4703, 7.6624) (23.5113, 7.6669) (23.5523, 7.6711) (23.5934, 7.675) (23.6346, 7.6786) (23.6759, 7.682) (23.7172, 7.6851) (23.7586, 7.688) (23.8, 7.6905) (23.8415, 7.6928) (23.8831, 7.6948) (23.9247, 7.6965) (23.9664, 7.698) (24.0082, 7.6992) (24.05, 7.7002) (24.0919, 7.7009) (24.1338, 7.7014) (24.1757, 7.7017) (24.2177, 7.7018) (24.2598, 7.7016) (24.3019, 7.7012) (24.344, 7.7005) (24.3862, 7.6997) (24.4284, 7.6986) (24.4707, 7.6973) (24.513, 7.6958) (24.5554, 7.6941) (24.5977, 7.6922) (24.6402, 7.69) (24.6826, 7.6877) (24.7251, 7.6852) (24.7677, 7.6825) (24.8102, 7.6795) (24.8528, 7.6764) (24.8954, 7.6731) (24.9381, 7.6696) (24.9808, 7.6659) (25.0235, 7.662) (25.0663, 7.6579) (25.109, 7.6536) (25.1518, 7.6492) (25.1947, 7.6445) (25.2375, 7.6397) (25.2804, 7.6347) (25.3233, 7.6295) (25.3662, 7.6242) (25.4092, 7.6186) (25.4522, 7.6129) (25.4952, 7.607) (25.5382, 7.6009) (25.5812, 7.5947) (25.6243, 7.5883) (25.6674, 7.5817) (25.7105, 7.5749) (25.7536, 7.568) (25.7967, 7.5609) (25.8399, 7.5536) (25.8744, 7.5477) (25.9003, 7.5431) (25.9176, 7.5401) (25.9263, 7.5385) knots 0 0 0 0 0 0 0.01428571 0.02857143 0.04285714 0.05714286 0.07142857 0.08571429 0.1 0.11428571 0.12857143 0.14285714 0.15714286 0.17142857 0.18571429 0.2 0.21428571 0.22857143 0.24285714 0.25714286 0.27142857 0.28571429 0.3 0.31428571 0.32857143 0.34285714 0.35714286 0.37142857 0.38571429 0.4 0.41428571 0.42857143 0.44285714 0.45714286 0.47142857 0.48571429 0.5 0.51428571 0.52857143 0.54285714 0.55714286 0.57142857 0.58571429 0.6 0.61428571 0.62857143 0.64285714 0.65714286 0.67142857 0.68571429 0.7 0.71428571 0.72857143 0.74285714 0.75714286 0.77142857 0.78571429 0.8 0.81428571 0.82857143 0.84285714 0.85714286 0.87142857 0.88571429 0.9 0.91428571 0.92857143 0.94285714 0.95714286 0.97142857 0.98571429 1 1 1 1 1 1
  line L49 (22.9886, 7.5724) -> (22.3464, 7.3611)
  arc A99 (21.0982, 7.9581) -> (22.3464, 7.3611) centre (22.0339, 8.311) ccw
  arc A100 (21.0982, 7.9581) -> (20.8276, 8.6415) centre (0, 0) ccw
  line L50 (0, 0) -> (3.1, 0) construction
  line L51 (2.6, -1.6882) -> (2.6, 1.6882)
  dimension "d309" = 0.5
  constraint coincident A0.centre A2.centre
  constraint coincident A0 L50.end
  constraint horizontal L50
  constraint coincident A0 L51.start
  constraint coincident A0 L51.end
  constraint perpendicular L50 L51
  measures "d309" distance of L50.end L51
extrude "Extrude3" add sketch "Sketch4" against normal blind 10 contours A0 L51 picked at (2.6718, -0.4326) bodies 3 in component "Spur Gear (25 teeth) encoder"
extrude "Extrude9" add sketch "Sketch1 (2)" against normal blind 5 from surface at -11 separate body contours A2 A5 A7 A9 A11 | A2 A5 A11 A20 | A2 A5 | A2 A5 A20 | A2 A11 A20 | A2 A11 | A2 A5 A7 A9 A11 A18 A20 | A5 A20 | A5 A11 A18 A20 A21 | A11 A20 | A2 A7 | A2 A7 | A2 A9 | A2 A9 | A18 A19 A20 A21 | A18 A19 A20 L8 A23 | A18 A19 A20 L11 A24 | A18 A19 A20 A21 | A15 A18 A19 A21 | A18 A21 | A18 A19 L8 L11 | A19 A20 A21 L8 A23 | A19 A20 A23 | A19 A20 A24 | A19 A20 A21 L11 A24 | A3 A15 A16 A17 A19 A21 | A19 L8 A23 | A19 A20 L8 L9 A23 | A19 A23 | A22 | A19 A20 L8 A23 | A20 A23 | A19 A20 L10 L11 A24 | A19 L11 A24 | A25 | A19 A20 L11 A24 | A19 A24 | A20 A24 | A12 A15 A19 | A3 A12 A15 A19 | A20 A21 L8 L11 | L8 A23 | A20 L8 A23 | L11 A24 | A20 L11 A24 | A3 A15 | A3 A15 A16 A17 | A12 A19 | A12 A19 | A3 A17 | A3 A17 | A3 A16 | A3 A16 | A4 | A6 | A8 | A10 | A13 | A14 makes body 4 in component "casing top"
extrude "Extrude10" add sketch "Sketch1 (2)" along normal blind 25 from surface at -11 contours A18 A19 L8 L11 | A19 A20 L8 L9 A23 | A19 A23 | A19 A20 L8 A23 | A20 A23 | A19 A20 L10 L11 A24 | A19 A20 L11 A24 | A19 A24 | A20 A24 | A20 A21 L8 L11 | L8 A23 | L11 A24 bodies 4 in component "casing top"
extrude "Extrude11" cut sketch "Sketch1 (2)" against normal blind 16 contours A22 | A25 bodies 4 in component "casing top"
fillet "Fillet6" radius 5 4 edges at (29.5818, 30, 1.5) (20.8182, 30, 1.5) (29.5818, -30, 1.5) (20.8182, -30, 1.5) on bodies 4 in component "casing top"
extrude "Extrude8" add sketch "Sketch1" against normal blind 5 contours A18 A21 bodies 1 in component "casing bottom"
extrude "Extrude9'" cut sketch "Sketch1" against normal blind 5 contours A22 | A25 bodies 1 in component "casing bottom"
component "casing bottom" placed x (1, 0, 0) y (0, 1, 0) z (0, 0, 1) at (0, 0, 0)
component "casing top" placed x (1, 0, 0) y (0, -1, 0) z (0, 0, -1) at (0, 0, 14.2302)
component "Spur Gear (25 teeth) motor" placed x (0.628586, 0.77774, 0) y (-0.77774, 0.628586, 0) z (0, 0, 1) at (0, 0, 0)
component "Spur Gear (25 teeth) encoder" placed x (0.628586, -0.77774, 0) y (0.77774, 0.628586, 0) z (0, 0, 1) at (50.4, 0, 0)
equation "d192_1_1_1 = 4 mm"
equation "d193_1_1_1 = -d192_1_1_1"
equation "d194_1_1_1 = 4 mm"
equation "d195_1_1_1 = -d194_1_1_1"
equation "d193_1_1_1_1 = -d192_1_1_1"
equation "d195_1_1_1_1 = -d194_1_1_1"
